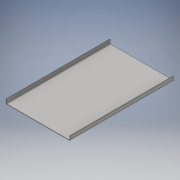
# Autodesk Inventor part: air tank mount
Saved by Autodesk Inventor 2016 (Build 200138000, 138)
## iProperties
Created: 2018-07-07
Part Number: air tank mount
Material: Generic
Document SubType Name: Sheet Metal
Designer: Kade
Density: 1 g/cm^3
Sheet Metal Rule: Default
Appearance: Default
Author: Kade
Autodesk Inventor part; units mm, degrees
ref_plane "YZ Plane" through (0, 0, 0) normal (1, 0, 0) x (0, 1, 0)
ref_plane "XZ Plane" through (0, 0, 0) normal (0, 1, 0) x (-1, 0, 0)
ref_plane "XY Plane" through (0, 0, 0) normal (0, 0, 1) x (1, 0, 0)
sketch "Sketch1" plane through (0, 0, 0) normal (0, 1, 0) x (-1, 0, 0)
  line L0 (0, 0) -> (-403.7076, 0)
  line L1 (-403.7076, 0) -> (-403.7076, -660.4)
  line L2 (-403.7076, -660.4) -> (0, -660.4)
  line L3 (0, -660.4) -> (0, 0)
  dimension "d0" = 403.7076
  dimension "d1" = 660.4
  measures "d0" distance of L2.end L1.end
  measures "d1" distance of L1.end L0.end
extrude "Plate1" add sketch "Sketch1" along normal blind 3.048
sketch "Sketch2" plane through (0, 3.048, 0) normal (0, 1, 0) x (1, 0, 0)
  line L0 (0, 0) -> (-25.4, 0)
  line L1 (-25.4, 0) -> (-25.4, 660.4)
  line L2 (-25.4, 660.4) -> (0, 660.4)
  line L3 (0, 660.4) -> (0, 0)
  line L4 (0, 0) -> (403.7076, 0) projected
  line L5 (403.7076, 0) -> (429.1076, 0)
  line L6 (429.1076, 0) -> (429.1076, 660.4)
  line L7 (429.1076, 660.4) -> (403.7076, 660.4)
  line L8 (403.7076, 660.4) -> (403.7076, 0)
  dimension "d3" = 25.4
  dimension "d4" = 25.4
  dimension "d22" = 660.4
  dimension "d23" = 660.4
  constraints: 16 end point, 4 parallel, 2 horizontal, 2 perpendicular
  measures "d3" distance of L1.end L2.end
  measures "d4" distance of L7.end L6.end
  measures "d22" distance of L5.end L6.end
  measures "d23" distance of L0.end L1.end
sheet face with bend "Face2" sketch "Sketch2" thickness 3.048 toward (0, -1, 0) bend radius 3.048 relief tear relief width 3.048 relief depth 1.524
bend "Bend1"
fold "Fold1" angle 90 bend radius 3.048 thickness 3.048 k factor 0.44 line from (0, 3.048, -660.4) to (0, 3.048, 0) line at bend centre moving side (-1, 0, 0) folds toward (0, 1, 0)
fold "Fold2" angle 90 bend radius 3.048 thickness 3.048 k factor 0.44 line from (403.7076, 3.048, -660.4) to (403.7076, 3.048, 0) line at bend centre moving side (1, 0, 0) folds toward (0, 1, 0)
equation "\"d10\" = BendReliefWidth"
equation "\"d11\" = BendReliefDepth"
equation "\"d12\" = MinimumRemnant"
equation "\"d13\" = BendRadius"
equation "\"d15\" = BendRadius"
equation "\"d16\" = BendReliefWidth"
equation "\"d17\" = BendReliefDepth"
equation "\"d18\" = MinimumRemnant"
equation "\"d19\" = BendRadius"
equation "\"d21\" = BendRadius"
equation "\"d5\" = BendRadius"
equation "\"d6\" = BendReliefWidth"
equation "\"d8\" = MinimumRemnant"
equation "\"d7\" = BendReliefDepth"
equation "\"d9\" = BendRadius"
equation "\"BendRadius\" = Thickness"
equation "\"BendReliefWidth\" = Thickness"
equation "\"BendReliefDepth\" = 0.5 * Thickness"
equation "\"CornerReliefSize\" = 4 * Thickness"
equation "\"MinimumRemnant\" = 2 * Thickness"
equation "\"TransitionRadius\" = BendRadius"
equation "\"JacobiRadiusSize\" = Thickness"
equation "\"GapSize\" = Thickness"
equation "\"d2\" = BendRadius"
equation "\"Thickness\" = 3.048"
body "Solid1"
